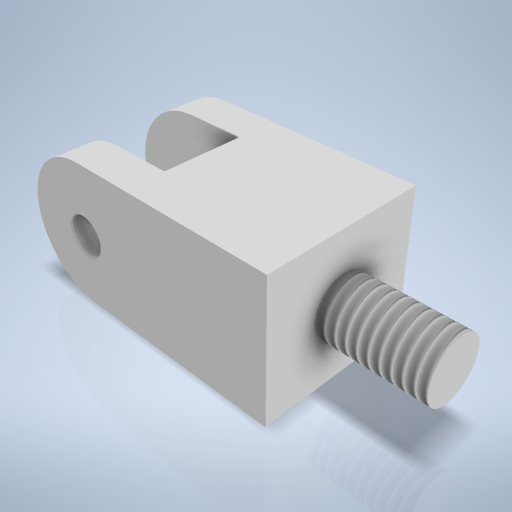
# Autodesk Inventor part: 25
Saved by Autodesk Inventor 2024.2 (Build 282272000, 272)
## iProperties
Created: 2024-05-15
Part Number: 25
Material: Generisch
Document SubType Name: Modeling
Designer: Fabri
Density: 1 g/cm^3
Appearance: Vorgabe
Author: Fabri
Autodesk Inventor part; units mm, degrees
ref_plane "YZ Plane" through (0, 0, 0) normal (1, 0, 0) x (0, 1, 0)
ref_plane "XZ Plane" through (0, 0, 0) normal (0, 1, 0) x (-1, 0, 0)
ref_plane "XY Plane" through (0, 0, 0) normal (0, 0, 1) x (1, 0, 0)
sketch "Skizze1" plane through (0, 0, 0) normal (0, 1, 0) x (-1, 0, 0)
  line L0 (0, 3.5) -> (14, 3.5)
  line L1 (14, 3.5) -> (14, -3.5)
  line L2 (14, -3.5) -> (0, -3.5)
  line L3 (0, -3.5) -> (0, 3.5)
  point P0 (0, 0)
  point P1 (0, 0)
  dimension "d0" = 7
  dimension "d1" = 14
  constraints: 8 end point, 2 parallel, 1 coincident, 1 horizontal, 1 midpoint, 1 perpendicular
  measures "d0" distance between parallel lines of L2 L0
  measures "d1" distance between parallel lines of L3 L1
extrude "Extrusion1" add sketch "Skizze1" along normal blind 8
fillet "Rundung1" radius 3.5 2 edges at (-14, 4, -3.5) (-14, 4, 3.5)
sketch "Skizze2" plane through (0, 8, 0) normal (0, 1, 0) x (1, 0, 0)
  arc A0 (-10.5, 3.5) -> (-10.5, -3.5) centre (-10.5, 0) ccw projected
  point P0 (0, 0)
  constraints: 1 coincident
hole "Bohrung1" at (-10.5, 8, 0) direction (0, -1, 0) diameter 2 depth 8
sketch "Skizze3" plane through (0, 0, -3.5) normal (0, 0, -1) x (-1, 0, 0)
  line L0 (7.5, 6) -> (16, 6)
  line L1 (16, 6) -> (16, 2)
  line L2 (16, 2) -> (7.5, 2)
  line L3 (7.5, 2) -> (7.5, 6)
  line L4 (14, 0) -> (14, 8) projected
  line L5 (0, 0) -> (0, 8) projected
  point P0 (7.5, 4)
  point P1 (0, 4)
  point P2 (11.75, 2)
  point P3 (16, 4)
  dimension "d12" = 6.5
  dimension "d13" = 4
  dimension "d14" = 2
  constraints: 8 end point, 4 midpoint, 2 parallel, 1 horizontal, 1 horizontal alignment, 1 perpendicular
  measures "d12" distance between parallel lines of L3 L4
  measures "d13" distance from line of point (11.75, 2) L0
  measures "d14" distance from line of L4 point (16, 4)
extrude "Extrusion2" cut sketch "Skizze3" against normal up to surface (7 mm away)
sketch "Skizze4" plane through (0, 0, 3.5) normal (1, 0, 0) x (0, 0, -1)
  circle A0 centre (3.5, 4) radius 1.5
  line L0 (7, 0) -> (7, 8) projected
  line L1 (0, 0) -> (7, 0) projected
  point P0 (3.5, 0)
  point P1 (7, 4)
  point P2 (3.5, 0)
  dimension "d17" = 3
  constraints: 2 midpoint, 1 centre point, 1 horizontal alignment, 1 vertical alignment
  measures "d17" diameter of A0
extrude "Extrusion3" add sketch "Skizze4" along normal blind 5
thread "Gewinde1" size "M3x0.5" class "6g" standard "ISO Metric profile" length 18
